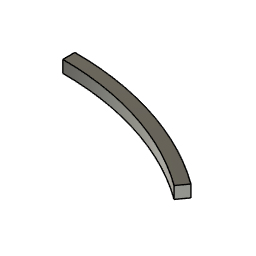
Boundary_Part (Autodesk Fusion 360 design; units mm, degrees)
Autodesk Fusion 360 part; units mm, degrees
sketch "Sketch1" plane through (0, 0, 0) normal (0, 0, 1) x (1, 0, 0)
  circle A0 centre (0, 0) radius 350
  circle A1 centre (0, 0) radius 365
  line L0 (0, 0) -> (0, 365)
  line L1 (0, 0) -> (-214.5416, 295.2912)
  line L2 (0, 0) -> (-347.1356, 112.7912)
  line L3 (0, 0) -> (-347.1356, -112.7912)
  line L4 (0, 0) -> (-214.5416, -295.2912)
  line L5 (0, 0) -> (0, -365)
  line L6 (0, 0) -> (214.5416, -295.2912)
  line L7 (0, 0) -> (347.1356, -112.7912)
  line L8 (0, 0) -> (347.1356, 112.7912)
  line L9 (0, 0) -> (214.5416, 295.2912)
  dimension "d1" = 700
  dimension "d2" = 15
  dimension "d4" = 360
  constraint coincident A0.centre A1.centre
  constraint coincident A1 L0.end
  constraint vertical L0
  measures "d1" diameter of A0
extrude "Extrude1" add sketch "Sketch1" along normal blind 15 contours A0 A1 L0 L9
